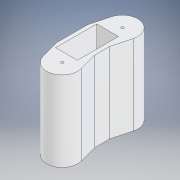
# Autodesk Inventor part: TA001
Saved by Autodesk Inventor 2017 SP1 (Build 210196100, 196)
## iProperties
Created: 2017-09-22
Part Number: TA001
Material: ABS Plastic
Document SubType Name: Modeling
Designer: Zach
Density: 1.06 g/cm^3
Appearance: CR White
Author: Zach
Autodesk Inventor part; units mm, degrees
ref_plane "YZ Plane" through (0, 0, 0) normal (1, 0, 0) x (0, 1, 0)
ref_plane "XZ Plane" through (0, 0, 0) normal (0, 1, 0) x (-1, 0, 0)
ref_plane "XY Plane" through (0, 0, 0) normal (0, 0, 1) x (1, 0, 0)
sketch "Sketch2" plane through (0, 0, 0) normal (0, 1, 0) x (-1, 0, 0)
  circle A0 centre (0, 0) radius 80 construction
  line L0 (77.2741, 20.7055) -> (103.156, -75.8871)
  line L1 (-77.2741, -20.7055) -> (-51.3922, -117.2981)
  line L2 (103.156, -75.8871) -> (-51.3922, -117.2981) construction
  line L3 (103.156, -75.8871) -> (103.156, -235.8871)
  line L4 (103.156, -235.8871) -> (-51.3922, -194.476) construction
  line L5 (-51.3922, -117.2981) -> (-51.3922, -194.476)
  circle A1 centre (0, -311.7741) radius 80 construction
  line L6 (-51.3922, -194.476) -> (-77.2741, -291.0686)
  line L7 (103.156, -235.8871) -> (77.2741, -332.4796)
  arc A2 (77.2741, 20.7055) -> (-77.2741, -20.7055) centre (0, 0) ccw
  arc A3 (-77.2741, -291.0686) -> (77.2741, -332.4796) centre (0, -311.7741) ccw
  circle A4 centre (0, 0) radius 7
  circle A5 centre (0, -311.7741) radius 7
  line L8 (83.156, -49.3871) -> (-29.844, -49.3871)
  line L9 (-29.844, -49.3871) -> (-29.844, -262.3871)
  line L10 (-29.844, -262.3871) -> (83.156, -262.3871)
  line L11 (83.156, -262.3871) -> (83.156, -49.3871)
  point P0 (103.156, -155.8871)
  point P1 (83.156, -155.8871)
  dimension "d0" = 160
  dimension "d1" = 100
  dimension "d2" = 100
  dimension "d3" = 160
  dimension "d4" = 160
  dimension "d5" = 160
  dimension "d6" = 75
  dimension "d7" = 75
  dimension "d8" = 160
  dimension "d9" = 100
  dimension "d10" = 100
  dimension "d11" = 14
  dimension "d12" = 14
  dimension "d13" = 113
  dimension "d14" = 213
  dimension "d15" = 20
  constraints: 24 end point, 8 point on circle, 8 tangent, 6 centre point, 3 coincident, 2 midpoint, 2 parallel, 1 horizontal, 1 horizontal alignment, 1 perpendicular, 1 vertical
  measures "d0" diameter of A0
  measures "d1" distance of L0.end L0.start
  measures "d2" distance of L1.end L1.start
  measures "d3" distance of L0.end L1.end
  measures "d4" distance of L0.end L3.end
  measures "d5" distance of L3.end L4.end
  measures "d6" angle of L3 L2
  measures "d7" angle of L3 L4
  measures "d8" diameter of A1
  measures "d9" distance of L4.end L6.end
  measures "d10" distance of L3.end L7.end
  measures "d11" diameter of A4
  measures "d12" diameter of A5
  measures "d13" distance of L10.end L9.end
  measures "d14" distance of L9.end L8.end
  measures "d15" distance between parallel lines of L3 L11
extrude "Extrusion1" add sketch "Sketch2" along normal blind 415
sketch "Sketch4" plane through (-103.156, 0, -235.8871) normal (-1, 0, 0) x (0, 0, 1)
  line L0 (-82.8871, 415) -> (-68.8871, 415) construction
  line L1 (228.8871, 415) -> (242.8871, 415) construction
  line L2 (242.8871, 0) -> (228.8871, 0) construction
  line L3 (-82.8871, 415) -> (-68.8871, 415) construction
  line L4 (-68.8871, 0) -> (-82.8871, 0) construction
  line L5 (-82.8871, 415) -> (-82.8871, 0) construction
  line L6 (-68.8871, 0) -> (-68.8871, 415) construction
  line L7 (228.8871, 415) -> (228.8871, 0) construction
  line L8 (228.8871, 0) -> (228.8871, 415) construction
  line L9 (242.8871, 0) -> (242.8871, 415) construction
  line L10 (215.1815, 0) -> (315.8871, 0) construction
  line L11 (-85.8871, 10) -> (-65.8871, 10)
  line L12 (-65.8871, 10) -> (-65.8871, 40)
  line L13 (-65.8871, 40) -> (-85.8871, 40)
  line L14 (-85.8871, 40) -> (-85.8871, 10)
  line L15 (-85.8871, 80) -> (-65.8871, 80)
  line L16 (-65.8871, 80) -> (-65.8871, 110)
  line L17 (-65.8871, 110) -> (-85.8871, 110)
  line L18 (-85.8871, 110) -> (-85.8871, 80)
  line L19 (225.8871, 10) -> (245.8871, 10)
  line L20 (245.8871, 10) -> (245.8871, 40)
  line L21 (245.8871, 40) -> (225.8871, 40)
  line L22 (225.8871, 40) -> (225.8871, 10)
  line L23 (225.8871, 80) -> (245.8871, 80)
  line L24 (245.8871, 80) -> (245.8871, 110)
  line L25 (245.8871, 110) -> (225.8871, 110)
  line L26 (225.8871, 110) -> (225.8871, 80)
  point P0 (235.8871, 0)
  point P1 (256.5926, 0)
  point P2 (-75.8871, 10)
  point P3 (-75.8871, 0)
  point P4 (-75.8871, 80)
  point P5 (-75.8871, 40)
  point P6 (235.8871, 80)
  point P7 (235.8871, 0)
  point P8 (235.8871, 10)
  dimension "d27" = 20
  dimension "d28" = 30
  dimension "d29" = 10
  dimension "d30" = 20
  dimension "d31" = 30
  dimension "d32" = 40
  dimension "d33" = 20
  dimension "d34" = 30
  dimension "d35" = 20
  dimension "d36" = 30
  constraints: 40 end point, 9 equal length, 7 midpoint, 5 perpendicular, 4 horizontal, 4 vertical alignment, 2 horizontal alignment, 1 vertical
  measures "d27" distance of L13.end L12.end
  measures "d28" distance of L12.end L11.end
  measures "d29" distance from line of point (-75.887, 0) L11
  measures "d30" distance of L17.end L16.end
  measures "d31" distance of L16.end L15.end
  measures "d32" distance between parallel lines of L13 L15
  measures "d33" distance of L21.end L20.end
  measures "d34" distance of L20.end L19.end
  measures "d35" distance of L25.end L24.end
  measures "d36" distance of L24.end L23.end
extrude "Extrusion3" cut sketch "Sketch4" against normal blind 113.156
body "Solid1"
